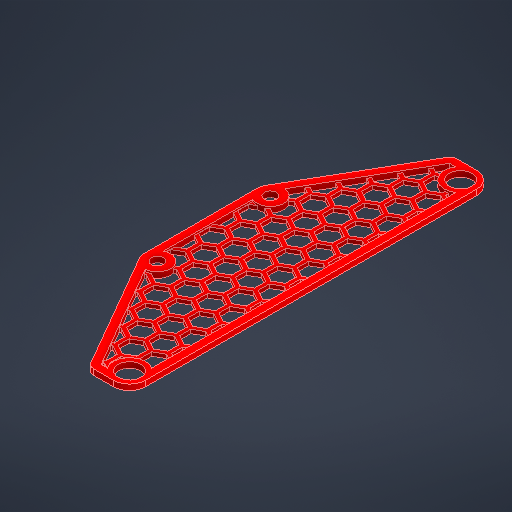
# Autodesk Inventor part: UpperSomething
Saved by Autodesk Inventor 2027 (Build 310192000, 192)
## iProperties
Created: 2026-09-26
Part Number: UpperSomething
Material: Všeobecné
Document SubType Name: Modeling
Designer: Vadim
Density: 1 g/cm^3
Appearance: Výchozí
Author: Vadim
Autodesk Inventor part; units mm, degrees
ref_plane "YZ Plane" through (0, 0, 0) normal (1, 0, 0) x (0, 1, 0)
ref_plane "XZ Plane" through (0, 0, 0) normal (0, 1, 0) x (-1, 0, 0)
ref_plane "XY Plane" through (0, 0, 0) normal (0, 0, 1) x (1, 0, 0)
sketch "Náčrt1" plane through (0, 0, 0) normal (0, 1, 0) x (-1, 0, 0)
  line L0 (29.315, 0) -> (29.315, 15.9378)
  line L1 (29.315, 15.9378) -> (11.2658, 47.2)
  line L2 (9.5337, 48.2) -> (0, 48.2)
  line L3 (0, 48.2) -> (0, 0)
  line L4 (29.315, 0) -> (0, 0)
  circle A0 centre (4.3, 43.9) radius 2.8
  circle A1 centre (4.3, 43.9) radius 4.3
  circle A2 centre (25.815, 15) radius 1.5
  circle A3 centre (25.815, 15) radius 3.5
  line L5 (25.815, 15) -> (17.9229, 15)
  line L6 (27.315, 11.8377) -> (27.315, 0)
  line L7 (9.5337, 46.2) -> (25.5329, 18.4886)
  line L8 (2, 0) -> (2, 40.2668)
  line L9 (7.9332, 46.2) -> (9.5337, 46.2)
  arc A4 (11.2658, 47.2) -> (9.5337, 48.2) centre (9.5337, 46.2) ccw
  point P0 (10.6884, 48.2)
  point P1 (29.315, 15)
  point P2 (28.8461, 16.75)
  point P3 (4.3, 48.2)
  point P4 (0, 43.9)
  dimension "d0" = 5.6
  dimension "d1" = 43.9
  dimension "d3" = 3
  dimension "d4" = 2
  dimension "d8" = 21.515
  dimension "d10" = 60
  dimension "d12" = 2
  dimension "d13" = 2
  dimension "d14" = 2
  dimension "d15" = 2
  dimension "d18" = 2
  dimension "d48" = 1.5
  dimension "d51" = 15
  constraints: 20 end point, 6 point on circle, 6 point on line, 6 tangent, 5 centre point, 3 perpendicular, 2 horizontal, 2 parallel, 1 coincident
  measures "d0" diameter of A0
  measures "d1" distance from line of L4 A0.centre
  measures "d3" diameter of A2
  measures "d4" radial gap between concentric circles of A2 A3
  measures "d8" horizontal distance of A0.centre L5.start
  measures "d10" angle of L1 L5
  measures "d12" distance between parallel lines of L1 L7
  measures "d13" distance between parallel lines of L3 L8
  measures "d14" distance between parallel lines of L2 L9
  measures "d15" distance between parallel lines of L0 L6
  measures "d18" radius of A4
  measures "d48" radial gap between concentric circles of A1 A0
  measures "d51" distance from line of L5.start L4
extrude "Vysunutí1" add sketch "Náčrt1" along normal blind 1.5 contours L4 L6 A3 L0 | A3 | A3 L7 L9 A1 L2 A4 L1 | L4 L3 A1 L8 | A1 | A0 | A2
sketch "Náčrt2" plane through (0, 1.5, 0) normal (0, 1, 0) x (1, 0, 0)
  arc A0 (-2, -40.2668) -> (-7.9332, -46.2) centre (-4.3, -43.9) ccw projected
  arc A1 (-25.5329, -18.4886) -> (-27.315, -11.8377) centre (-25.815, -15) ccw projected
  point P0 (0, 0)
  point P1 (-4.3, -43.9)
  constraints: 2 coincident
hole "Díra1" at (-4.3, 1.5, 43.9) direction (0, -1, 0) diameter 6 end through all
sketch "Náčrt4" plane through (0, 1.5, 0) normal (0, 1, 0) x (1, 0, 0)
  arc A0 (-25.5329, -18.4886) -> (-27.315, -11.8377) centre (-25.815, -15) ccw projected
  point P0 (0, 0)
  constraints: 1 coincident
hole "Díra2" at (-25.815, 1.5, 15) direction (0, -1, 0) diameter 3.2 end through all
extrude "Vysunutí2" add sketch "Náčrt1" along normal blind 1 separate body contours L4 L8 A1 L9 L7 A3 L6
mirror "Zrcadlit1" about plane through (-27.315, 0, 0) normal (0, 0, -1) bodies 1 2
sketch "Náčrt3" plane through (0, 1, 0) normal (0, 1, 0) x (1, 0, 0)
  arc A0 (-2, -40.2668) -> (-7.9332, -46.2) centre (-4.3, -43.9) ccw projected
  line L0 (-2, -40.2668) -> (-2, 40.2668) projected
  line L1 (-27.315, -11.8377) -> (-27.315, 11.8377) projected
  arc A1 (-25.5329, -18.4886) -> (-27.315, -11.8377) centre (-25.815, -15) ccw projected
  line L2 (-25.5329, -18.4886) -> (-9.5337, -46.2) projected
  line L3 (-9.5337, -46.2) -> (-7.9332, -46.2) projected
  line L4 (-17.5333, -32.3443) -> (-2.3155, 0.5581) construction
  line L5 (-26.2523, 1.0972) -> (-2, -40.2668) construction
  line L6 (-15.2318, -20.519) -> (-12.7318, -19.0756)
  line L7 (-12.7318, -19.0756) -> (-10.2318, -20.452)
  line L8 (-10.2318, -20.452) -> (-10.2318, -23.4058)
  line L9 (-10.2318, -23.4058) -> (-12.6735, -24.8155)
  line L10 (-12.6735, -24.8155) -> (-15.2318, -23.4069)
  line L11 (-15.2318, -23.4069) -> (-15.2318, -20.519)
  line L12 (-2, -40.2668) -> (-2, 0.5581) projected
  line L13 (-12.7318, -21.963) -> (-15.2318, -21.963) construction
  line L14 (-13.9526, -24.1112) -> (-12.7318, -21.963) construction
  arc A2 (-7.9332, 46.2) -> (-2, 40.2668) centre (-4.3, 43.9) ccw projected
  line L15 (-9.5337, 46.2) -> (-7.9332, 46.2) projected
  line L16 (-25.5329, 18.4886) -> (-9.5337, 46.2) projected
  arc A3 (-27.315, 11.8377) -> (-25.5329, 18.4886) centre (-25.815, 15) ccw projected
  point P0 (0, 0)
  dimension "d30" = 5
  dimension "d49" = 5
  dimension "d50" = 5
  constraints: 20 end point, 3 midpoint, 3 parallel, 2 point on line, 1 horizontal
  measures "d30" distance between parallel lines of L8 L11
  measures "d49" distance between parallel lines of L10 L7
  measures "d50" distance between parallel lines of L6 L9
extrude "Vysunutí3" cut sketch "Náčrt3" against normal through all contours L6 L7 L8 L9 L10 L11 bodies 2
pattern_linear "Obdélníkové pole1" count 16 spacing 6 along (1, 0, 0) count 26 spacing 6 along (-0.5, 0, -0.8660254) of "Vysunutí3" first direction both ways yes second direction both ways yes bodies 2
